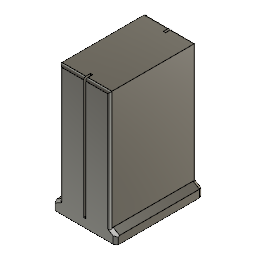
light-baffle (Autodesk Fusion 360 design; units mm, degrees)
Autodesk Fusion 360 part; units mm, degrees
note: some values were not read from the file. Chosen so that the rebuilt part matches the saved one: which pieces of a blend or face edit are solid.
sketch "Sketch1" plane through (0, 0, 0) normal (0, 0, 1) x (1, 0, 0)
  line L0 (0, 0) -> (14.6, 0)
  line L1 (14.6, 0) -> (14.6, 20)
  line L2 (14.6, 20) -> (0, 20)
  line L3 (0, 20) -> (0, 0)
  line L4 (1.5, 0) -> (1.5, 20)
  line L5 (13.1, 20) -> (13.1, 0)
  line L6 (7.3, 0) -> (7.3, 20) construction
  dimension "d68" = 20
  dimension "d69" = 14.6
  dimension "d71" = 5.8
  dimension "d72" = 5.8
  dimension "d92" = 0
  dimension "d93" = 0
  dimension "d94" = 0
  dimension "d95" = 0
  measures "d69" distance of L0.start
  measures "d71" distance of L5 L6
  measures "d72" distance of L4 L6
extrude "Extrude1" add sketch "Sketch1" along normal blind 30 contours L0 L2 L4 L5
extrude "Extrude2" add sketch "Sketch1" along normal blind 2.65 contours L0 L2 L3 L4 | L0 L1 L2 L5
chamfer "Chamfer1" distance 1.5 angle 30 2 edges at (14.6, 10, 2.65) (0, 10, 2.65) measured on face at (13.6, 6.6667, 2.65) measured on face at (0.5, 13.3333, 2.65)
sketch "Sketch2" plane through (0, 0, 30) normal (0, 0, 1) x (-1, 0, 0)
  line L0 (-1.5, 0) -> (-13.1, 0)
  line L1 (-13.1, 0) -> (-13.1, -20)
  line L2 (-13.1, -20) -> (-1.5, -20)
  line L3 (-1.5, -20) -> (-1.5, 0)
  line L4 (-3.1, -20) -> (-3.1, 0)
  line L5 (-11.5, -20) -> (-11.5, 0)
  line L6 (-1.5, -18.4) -> (-13.1, -18.4)
  line L7 (-1.5, -1.6) -> (-13.1, -1.6)
  line L8 (-7.05, -20) -> (-7.05, 0)
  line L9 (-7.55, -20) -> (-7.55, 0)
  line L10 (-7.3, -20) -> (-7.3, 0) construction
  dimension "d79" = 1.6
  dimension "d80" = 1.6
  dimension "d81" = 1.6
  dimension "d82" = 1.6
  dimension "d83" = 0.25
  dimension "d84" = 0.25
  measures "d79" distance of L3 L4
  measures "d80" distance of L1 L5
  measures "d81" distance of L0 L7
  measures "d82" distance of L2 L6
  measures "d83" distance of L8 L10
  measures "d84" distance of L9 L10
extrude "Extrude3" cut sketch "Sketch2" against normal blind 28 contours L0 L7 L8 L9 | L4 L6 L7 L8 | L6 L7 L8 L9 | L5 L6 L7 L9 | L2 L6 L8 L9
extrude "Extrude4" add sketch "Sketch2" against normal blind 1.5 contours L4 L6 L7 L8 | L6 L7 L8 L9 | L5 L6 L7 L9
fillet "Fillet1" radius 0.5 8 edges at (13.1, 20, 16.325) (1.5, 20, 16.325) (10.325, 20, 30) (4.275, 20, 30) (10.325, 0, 30) (4.275, 0, 30) (13.1, 0, 16.325) (1.5, 0, 16.325)
chamfer "Chamfer2" distance 0.75 angle 30 8 edges at (13.6, 0, 2.3613) (1, 0, 2.3613) (0, 0, 0.892) (14.6, 0, 0.892) (13.6, 20, 2.3613) (14.6, 20, 0.892) (1, 20, 2.3613) (0, 20, 0.892) measured on face at (14.1001, 6.6667, 2.0728) measured on face at (0.4999, 13.3333, 2.0728) measured on face at (0, 13.3333, 0.5947) measured on face at (9.2397, 0, 11.4823) measured on face at (14.1001, 6.6667, 2.0728) measured on face at (14.6, 6.6667, 0.5947) measured on face at (0.4999, 13.3333, 2.0728) measured on face at (9.2397, 20, 11.4823)
equation "d71 = ( 11.6 / 2 ) * 1 mm"
equation "d72 = ( 11.6 / 2 ) * 1 mm"
